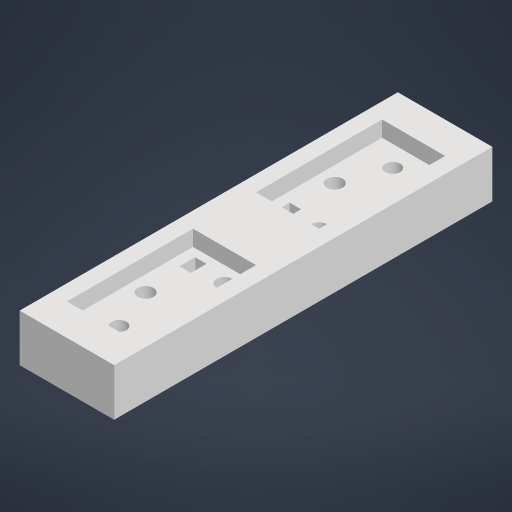
# Autodesk Inventor part: ExtendedSlottedCarrier
Saved by Autodesk Inventor 2024.1 (Build 281209000, 209)
## iProperties
Created: 2023-08-17
Part Number: ExtendedSlottedCarrier
Material: Generic
Document SubType Name: Modeling
Designer: Eleanor
Density: 1 g/cm^3
Appearance: Default
Author: Eleanor
Autodesk Inventor part; units mm, degrees
ref_plane "YZ Plane" through (0, 0, 0) normal (1, 0, 0) x (0, 1, 0)
ref_plane "XZ Plane" through (0, 0, 0) normal (0, 1, 0) x (-1, 0, 0)
ref_plane "XY Plane" through (0, 0, 0) normal (0, 0, 1) x (1, 0, 0)
sketch "Sketch1" plane through (0, 0, 0) normal (0, 1, 0) x (-1, 0, 0)
  line L0 (-6.35, 12.7) -> (6.35, 12.7)
  line L1 (6.35, 12.7) -> (6.35, -12.7)
  line L2 (6.35, -12.7) -> (-6.35, -12.7)
  line L3 (-6.35, -12.7) -> (-6.35, 12.7)
  line L4 (-6.35, 12.7) -> (6.35, -12.7) construction
  line L5 (6.35, 12.7) -> (-6.35, -12.7) construction
  line L6 (-9.525, 19.05) -> (9.525, 19.05)
  line L7 (9.525, 19.05) -> (9.525, -19.05)
  line L8 (9.525, -19.05) -> (-9.525, -19.05)
  line L9 (-9.525, -19.05) -> (-9.525, 19.05)
  line L10 (-9.525, 19.05) -> (9.525, -19.05) construction
  line L11 (9.525, 19.05) -> (-9.525, -19.05) construction
  line L12 (6.35, 15.875) -> (9.525, 15.875)
  line L13 (6.35, 15.875) -> (-9.525, 15.875)
  point P0 (0, 0)
  dimension "d0" = 12.7
  dimension "d1" = 25.4
  constraints: 28 end point, 4 midpoint, 4 parallel, 4 point on line, 3 perpendicular, 2 horizontal
  measures "d0" distance of L1.end L2.end
  measures "d1" distance of L0.end L1.end
extrude "Extrusion1" add sketch "Sketch1" along normal blind 3.175
sketch "Sketch2" plane through (0, 3.175, 0) normal (0, 1, 0) x (1, 0, 0)
  circle A0 centre (3.175, -9.525) radius 1.5875
  circle A1 centre (-3.175, 0) radius 1.5875
  circle A2 centre (0, 8.5298) radius 1.5
  line L0 (-4.318, -7.9375) -> (-2.032, -7.9375)
  line L1 (-2.032, -7.9375) -> (-2.032, -11.1125)
  line L2 (-2.032, -11.1125) -> (-4.318, -11.1125)
  line L3 (-4.318, -11.1125) -> (-4.318, -7.9375)
  line L4 (-4.318, -7.9375) -> (-2.032, -11.1125) construction
  line L5 (-2.032, -7.9375) -> (-4.318, -11.1125) construction
  line L6 (-9.525, 19.05) -> (-9.525, -19.05) projected
  line L7 (9.525, -19.05) -> (-9.525, -19.05)
  line L8 (-9.525, -19.05) -> (-9.525, 19.05)
  line L9 (-9.525, 19.05) -> (9.525, 19.05)
  line L10 (9.525, 19.05) -> (9.525, -19.05)
  line L11 (9.525, -19.05) -> (-9.525, 19.05) construction
  line L12 (-9.525, -19.05) -> (9.525, 19.05) construction
  point P0 (0, 0)
  point P1 (0, 0)
  dimension "d4" = 3.175
  dimension "d5" = 3.175
  dimension "d6" = 3
  dimension "d8" = 3.175
  constraints: 24 end point, 4 parallel, 3 centre point, 2 horizontal, 2 midpoint, 2 perpendicular
  measures "d4" diameter of A0
  measures "d5" diameter of A1
  measures "d6" diameter of A2
  measures "d8" distance of L2.end L0.start
extrude "Extrusion2" add sketch "Sketch2" along normal blind 3.175
sketch "Sketch3" plane through (0, 6.35, 0) normal (0, 1, 0) x (1, 0, 0)
  line L0 (-9.525, 19.05) -> (-9.525, -19.05) projected
  line L1 (9.525, -19.05) -> (-9.525, -19.05)
  line L2 (-9.525, -19.05) -> (-9.525, 19.05)
  line L3 (-9.525, 19.05) -> (9.525, 19.05)
  line L4 (9.525, 19.05) -> (9.525, -19.05)
  line L5 (9.525, -19.05) -> (-9.525, 19.05) construction
  line L6 (-9.525, -19.05) -> (9.525, 19.05) construction
  line L7 (6.35, -12.7) -> (-6.35, -12.7)
  line L8 (-6.35, -12.7) -> (-6.35, 12.7)
  line L9 (-6.35, 12.7) -> (6.35, 12.7)
  line L10 (6.35, 12.7) -> (6.35, -12.7)
  line L11 (6.35, -12.7) -> (-6.35, 12.7) construction
  line L12 (-6.35, -12.7) -> (6.35, 12.7) construction
  point P0 (0, 0)
  constraints: 24 end point, 4 midpoint, 4 parallel, 2 horizontal, 2 perpendicular
extrude "Extrusion3" add sketch "Sketch3" along normal blind 3.175
mirror "Mirror3" about plane through (-9.525, 0, 19.05) normal (0, 0, 1) of "Extrusion1", "Extrusion2", "Extrusion3"
body "Solid1"
